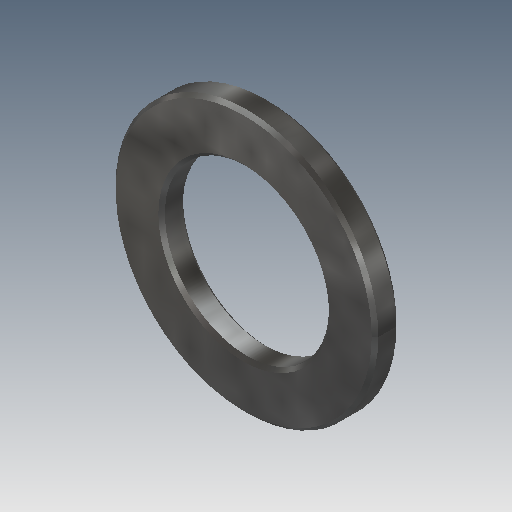
# Autodesk Inventor part: Separador16mm
Saved by Autodesk Inventor 2018 (Build 220112000, 112)
## iProperties
Created: 2016-06-29
Part Number: Separador16mm
Material: Steel
Document SubType Name: Modeling
Designer: YeseF
Density: 7.85 g/cm^3
Appearance: Steel Galvanized
Mass: 1.41705 g
Surface Area: 3.48427 cm^2
Volume: 0.180516 cm^3
Author: YeseF
Autodesk Inventor part; units mm, degrees
ref_plane "YZ Plane" through (0, 0, 0) normal (1, 0, 0) x (0, 1, 0)
ref_plane "XZ Plane" through (0, 0, 0) normal (0, 1, 0) x (-1, 0, 0)
ref_plane "XY Plane" through (0, 0, 0) normal (0, 0, 1) x (1, 0, 0)
sketch "Sketch1" plane through (0, 0, 0) normal (0, 0, 1) x (1, 0, 0)
  circle A0 centre (0, 0) radius 5
  circle A1 centre (0, 0) radius 8
  dimension "d0" = 10
  dimension "d1" = 16
  constraints: 2 centre point, 2 coincident
  measures "d0" diameter of A0
  measures "d1" diameter of A1
extrude "Extrusion1" add sketch "Sketch1" along normal blind 1.5
chamfer "Chamfer1" distance 0.2 angle 45 4 edges at (-8, 0, 1.5) (-5, 0, 1.5) (-5, 0, 0) (-8, 0, 0)
body "Solid1"
